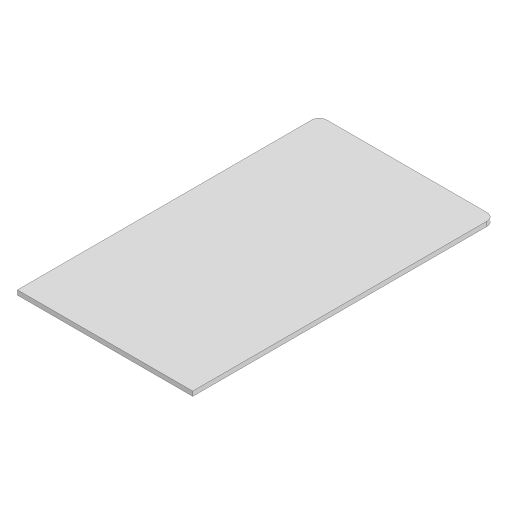
# Autodesk Inventor part: PMMA_lid_long
Saved by Autodesk Inventor 2023 (Build 270158000, 158)
## iProperties
Created: 2026-05-29
Part Number: PMMA_lid_long
Material: Generic
Document SubType Name: Modeling
Designer: ferrerx
Density: 1 g/cm^3
Appearance: Default
Author: ferrerx
Autodesk Inventor part; units mm, degrees
ref_plane "YZ Plane" through (0, 0, 0) normal (1, 0, 0) x (0, 1, 0)
ref_plane "XZ Plane" through (0, 0, 0) normal (0, 1, 0) x (-1, 0, 0)
ref_plane "XY Plane" through (0, 0, 0) normal (0, 0, 1) x (1, 0, 0)
sketch "Sketch1" plane through (0, 0, 0) normal (0, 1, 0) x (-1, 0, 0)
  line L0 (-57.5, 124) -> (57.5, 124)
  line L1 (57.5, 124) -> (57.5, -124)
  line L2 (57.5, -124) -> (-57.5, -124)
  line L3 (-57.5, -124) -> (-57.5, 124)
  line L4 (-57.5, 124) -> (57.5, -124) construction
  line L5 (57.5, 124) -> (-57.5, -124) construction
  point P0 (0, 0)
  dimension "d0" = 248
  dimension "d1" = 115
  constraints: 12 end point, 2 midpoint, 2 parallel, 1 horizontal, 1 perpendicular
  measures "d0" distance of L0.end L1.end
  measures "d1" distance of L0.start L0.end
extrude "Extrusion1" add sketch "Sketch1" along normal blind 3
fillet "Fillet1" radius 5 4 edges at (57.5, 1.5, 124) (57.5, 1.5, -124) (-57.5, 1.5, 124) (-57.5, 1.5, -124)
sketch "Sketch2" plane through (0, 3, 0) normal (0, 1, 0) x (1, 0, 0)
  line L0 (-57.5, -124) -> (57.5, -124)
  line L1 (57.5, -124) -> (57.5, -74)
  line L2 (57.5, -74) -> (-57.5, -74)
  line L3 (-57.5, -74) -> (-57.5, -124)
  line L4 (-52.5, -124) -> (52.5, -124) projected
  line L5 (57.5, -119) -> (57.5, 119) projected
  line L6 (-57.5, 119) -> (-57.5, -119) projected
  point P0 (0, 0)
  dimension "d5" = 50
  constraints: 8 end point, 3 collinear, 2 parallel, 1 horizontal, 1 perpendicular
  measures "d5" distance between parallel lines of L0 L2
extrude "Extrusion2" cut sketch "Sketch2" against normal blind 3
body "Solid1"
